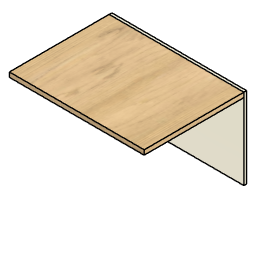
Camera mount v3 (Autodesk Fusion 360 design; units mm, degrees)
Autodesk Fusion 360 part; units mm, degrees
sketch "Sketch1" plane through (0, 0, 0) normal (0, 1, 0) x (1, 0, 0) in component "Shelf"
  line L0 (0, 0) -> (500, 0)
  line L1 (500, 0) -> (500, -17.3)
  line L2 (500, -17.3) -> (0, -17.3)
  line L3 (0, -17.3) -> (0, 0)
  line L4 (0, -17.3) -> (0, 282.7)
  line L5 (0, 282.7) -> (500, 282.7)
  line L6 (500, 282.7) -> (500, -17.3)
  dimension "d1" = 500
  dimension "d2" = 17.3
  dimension "d5" = 300
  constraint coincident L0.start L3.end
  constraint horizontal L0
  constraint perpendicular L0 L1
  constraint perpendicular L1 L2
  constraint perpendicular L0 L3
  constraint perpendicular L0 L4
  constraint perpendicular L1 L5
  constraint perpendicular L2 L6
  measures "d1" distance of L0.start L0.end
  measures "d2" distance of L0.end L1.end
  measures "d5" distance of L2.end L4.end
extrude "Extrude1" add sketch "Sketch1" against normal blind 370 contours L0 L1 L2 L3 L4 L6 makes body 1 in component "Shelf"
extrude "Extrude2" add sketch "Sketch1" along normal blind 10 separate body makes body 2 in component "Shelf"
sketch "Sketch2" plane through (0, 0, 0) normal (0, -1, 0) x (1, 0, 0) in component "Shelf"
  line L0 (0, -282.7) -> (500, -282.7)
  line L1 (500, -282.7) -> (500, 17.3)
  line L2 (500, 17.3) -> (0, 17.3)
  line L3 (0, 17.3) -> (0, -282.7)
  line L4 (0, 0) -> (500, 0)
  line L5 (500, 0) -> (0, 0)
  line L6 (236, 0) -> (236, -200)
  line L7 (236, -200) -> (264, -200)
  line L8 (264, -200) -> (264, 0)
  line L9 (250, -200) -> (250, 200) construction
  dimension "d8" = 200
  dimension "d9" = 28
  constraint coincident L5 L6.start
  constraint perpendicular L5 L6
  constraint perpendicular L6 L7
  constraint coincident L4 L8.end
  constraint perpendicular L4 L8
  constraint midpoint L7 L9.start
  constraint perpendicular L7 L9
  constraint midpoint L5 L9
  measures "d8" distance of L6.start L6.end
  measures "d9" distance of L6.end L7.end
extrude "Extrude3" add sketch "Sketch2" along normal blind 4 separate body contours L4 L5 L6 L7 L8 makes body 3 in component "Shelf"
sketch "Sketch3" plane through (0, -4, 0) normal (0, -1, 0) x (1, 0, 0) in component "Shelf"
  line L0 (264, -200) -> (264, 0)
  line L1 (264, 0) -> (236, 0)
  line L2 (236, 0) -> (236, -200)
  line L3 (236, -200) -> (264, -200)
  line L4 (236, -4) -> (264, -4)
  dimension "d12" = 4
  constraint coincident L2 L4.start
  constraint coincident L0 L4.end
  constraint perpendicular L0 L4
  measures "d12" distance of L1 L4
extrude "Extrude4" add sketch "Sketch3" along normal blind 280 contours L0 L1 L2 L4 bodies 3 in component "Shelf"
ref_plane "WorkPlane1" through (250, 0, 0) normal (1, 0, 0) x (0, 1, 0) in component "Shelf"
sketch "Sketch4" plane through (250, 0, 0) normal (1, 0, 0) x (0, 1, 0) in component "Shelf"
  line L0 (-4, -155) -> (-245.6505, -4)
  line L1 (-4, -4) -> (-284, -4)
  line L2 (-4, -4) -> (-4, -200)
  line L3 (-4, -155) -> (-186.4554, -155) construction
  line L4 (0, 0) -> (-370, 0) construction
  line L5 (-207.9089, -4) -> (-4, -131.4164)
  line L6 (-4, -131.4164) -> (-4, -155)
  line L7 (-207.9089, -4) -> (-245.6505, -4)
  dimension "d16" = 32
  dimension "d17" = 155
  dimension "d19" = 20
  constraint coincident L0.end L1
  constraint coincident L0.start L2
  constraint perpendicular L2 L3
  constraint coincident L1 L5.start
  constraint coincident L2 L5.end
  constraint parallel L0 L5
  measures "d16" angle of L0 L3
  measures "d17" distance of L0.start L4
  measures "d19" distance of L0 L5
extrude "Extrude5" add sketch "Sketch4" along normal mid plane 4.4 contours L0 L1 L2 L5 L6 L7 bodies 3 in component "Shelf"
sketch "Sketch1 (2)" plane through (247.8, 0, 0) normal (-1, 0, 0) x (0, -1, 0) in component "Mount"
  line L0 (207.9089, -4) -> (4, -131.4164)
  line L1 (4, -131.4164) -> (4, -155)
  line L2 (4, -155) -> (245.6505, -4)
  line L3 (245.6505, -4) -> (207.9089, -4)
  line L4 (0, 0) -> (0, -200)
  line L5 (0, -200) -> (4, -200)
  line L6 (4, -200) -> (4, -4)
  line L7 (4, -4) -> (284, -4)
  line L8 (284, -4) -> (284, 0)
  line L9 (284, 0) -> (0, 0)
  line L10 (4, -124.3414) -> (141.1258, -38.6557)
  line L11 (141.1258, -38.6557) -> (144.3053, -43.7439)
  dimension "d22" = 75
  dimension "d23" = 6
  constraint coincident L6 L10.start
  constraint parallel L0 L10
  constraint coincident L0 L11.end
  constraint perpendicular L0 L11
  measures "d22" distance of L0.start L11.end
  measures "d23" distance of L0 L10
sketch "Sketch5" plane through (0, -4, 0) normal (0, -1, 0) x (1, 0, 0) in component "Shelf"
  line L0 (247.8, -155) -> (247.8, -131.4164)
  line L1 (247.8, -131.4164) -> (252.2, -131.4164)
  line L2 (252.2, -131.4164) -> (252.2, -155)
  line L3 (252.2, -155) -> (247.8, -155)
  line L4 (264, -4) -> (236, -4)
  line L5 (236, -4) -> (236, -200)
  line L6 (236, -200) -> (264, -200)
  line L7 (264, -200) -> (264, -4)
  circle A0 centre (250, -188) radius 5
  line L8 (250, -155) -> (250, -197.5396) construction
  dimension "d31" = 10
  dimension "d32" = 33
  constraint midpoint L3 L8.start
  constraint perpendicular L3 L8
  constraint coincident A0.centre L8
  measures "d31" diameter of A0
  measures "d32" distance of L3 A0.centre
extrude "Extrude5'" add sketch "Sketch1 (2)" against normal blind 14.4 separate body contours L0 L6 L10 L11 makes body 4 in component "Mount"
sketch "Sketch6" plane through (262.2, 0, 0) normal (1, 0, 0) x (0, 1, 0) in component "Mount"
  line L0 (-4, -124.3414) -> (-141.1258, -38.6557)
  line L1 (-141.1258, -38.6557) -> (-144.3053, -43.7439)
  line L2 (-144.3053, -43.7439) -> (-4, -131.4164)
  line L3 (-4, -131.4164) -> (-4, -124.3414)
  line L4 (-4, -131.4164) -> (-4, -156.4164)
  line L5 (-4, -155) -> (-245.6505, -4)
  line L6 (-14, -148.7513) -> (-14, -176.9164)
  line L7 (-4, -200) -> (-4, -4)
  line L8 (-14, -176.9164) -> (-4, -176.9164)
  line L9 (-14, -148.7513) -> (-14, -125.1677)
  line L10 (-144.3053, -43.7439) -> (-155.9635, -62.401)
  line L11 (-155.9635, -62.401) -> (-14, -151.1097)
  dimension "d43" = 25
  dimension "d44" = 10
  dimension "d46" = 20.5
  dimension "d79" = 22
  constraint coincident L2.end L3.start
  constraint parallel L3 L4
  constraint coincident L5 L6.start
  constraint parallel L4 L6
  constraint coincident L7 L8.end
  constraint perpendicular L7 L8
  constraint coincident L2 L9.end
  constraint parallel L6 L9
  constraint coincident L1.end L2.start
  constraint perpendicular L5 L10
  constraint coincident L6 L11.end
  constraint perpendicular L10 L11
  measures "d43" distance of L2.end L4.end
  measures "d44" distance of L6 L7
  measures "d46" distance of L4.end L8.end
  measures "d79" distance of L1.end L10.end
extrude "Extrude6" add sketch "Sketch6" against normal blind 9.9 contours L2 L4 L5 L7 L9 | L4 L5 L6 L7 L8 bodies 4 in component "Mount"
sketch "Sketch7" plane through (0, -4, 0) normal (0, -1, 0) x (1, 0, 0) in component "Mount"
  line L0 (247.8, -155) -> (247.8, -131.4164)
  line L1 (247.8, -131.4164) -> (252.2, -131.4164)
  line L2 (252.2, -131.4164) -> (252.2, -155)
  line L3 (252.2, -155) -> (247.8, -155)
  line L4 (264, -4) -> (236, -4)
  line L5 (236, -4) -> (236, -200)
  line L6 (236, -200) -> (264, -200)
  line L7 (264, -200) -> (264, -4)
  circle A0 centre (250, -188) radius 3.5
  line L8 (250, -155) -> (250, -238.8329) construction
  line L9 (262.2, -176.9164) -> (252.3, -176.9164)
  line L10 (262.2, -176.9164) -> (262.2, -196.9164)
  line L11 (262.2, -196.9164) -> (237.8, -196.9164)
  line L12 (237.8, -196.9164) -> (237.8, -176.9164)
  line L13 (237.8, -176.9164) -> (252.3, -176.9164)
  dimension "d49" = 7
  dimension "d50" = 33
  dimension "d51" = 20
  constraint midpoint L3 L8.start
  constraint perpendicular L6 L8
  constraint coincident A0.centre L8
  constraint coincident L9.start L10.start
  constraint perpendicular L9 L10
  constraint perpendicular L10 L11
  constraint perpendicular L9 L12
  constraint coincident L9.end L13.end
  constraint perpendicular L8 L13
  constraint midpoint L8 L11
  measures "d49" diameter of A0
  measures "d50" distance of L3 A0.centre
  measures "d51" distance of L9.start L10.end
extrude "Extrude7" add sketch "Sketch7" along normal blind 6 contours L9 L10 L11 L12 L13 bodies 4 in component "Mount"
extrude "Extrude8" add 1 faces at (247.8, -50.7684, -99.8339) along direction (-1, 0, 0) blind 30 on bodies 4 bodies 4 in component "Mount"
sketch "Sketch8" plane through (217.8, 0, 0) normal (-1, 0, 0) x (0, -1, 0) in component "Mount"
  line L0 (141.1258, -38.6557) -> (4, -124.3414)
  line L1 (4, -124.3414) -> (4, -131.4164)
  line L2 (4, -131.4164) -> (144.3053, -43.7439)
  line L3 (144.3053, -43.7439) -> (141.1258, -38.6557)
  line L4 (104, -68.9295) -> (204, -68.9295) construction
  line L5 (104, -68.9295) -> (164, -68.9295)
  line L6 (164, -68.9295) -> (164, -143.9295)
  line L7 (104, -68.9295) -> (104, -143.9295)
  line L8 (104, -143.9295) -> (164, -143.9295)
  line L9 (154, -68.9295) -> (154, -165.7492) construction
  line L10 (4, -4) -> (4, -200)
  circle A0 centre (154, -133.9295) radius 3.25
  line L11 (144.3053, -43.7439) -> (164, -68.9295)
  line L12 (4, -131.4164) -> (4, -143.9295)
  line L13 (4, -143.9295) -> (104, -143.9295)
  dimension "d56" = 100
  dimension "d57" = 60
  dimension "d58" = 75
  dimension "d59" = 50
  dimension "d60" = 100
  dimension "d61" = 6.5
  dimension "d63" = 65
  constraint coincident L2 L4.start
  constraint horizontal L4
  constraint parallel L4 L5
  constraint perpendicular L4 L6
  constraint perpendicular L5 L7
  constraint perpendicular L6 L8
  constraint coincident L4 L9.start
  constraint perpendicular L8 L9
  constraint coincident L9 A0.centre
  constraint coincident L2.end L3.start
  constraint coincident L1.end L2.start
  constraint perpendicular L7 L13
  constraint perpendicular L12 L13
  measures "d56" distance of L4.start L4.end
  measures "d57" distance of L4.start L5.end
  measures "d58" distance of L5.end L6.end
  measures "d59" distance of L7 L9
  measures "d60" distance of L4.start L10
  measures "d61" diameter of A0
  measures "d63" distance of L5 A0.centre
extrude "Extrude9" add sketch "Sketch8" against normal blind 13 contours L2 L5 L11 | L2 L7 L10 L12 L13 | L5 L6 L7 L8 bodies 4 in component "Mount"
extrude "Extrude10" add 1 faces at (259.287, -10, -187.1037) along direction (0, -1, 0) blind 4 on bodies 4 bodies 4 in component "Mount"
hole "Hole1" at (250, -14, -188) direction (0, 1, 0) diameter 7 depth 10 tip angle 118 countersink diameter 10 countersink angle 80 bodies 4 in component "Mount"
fillet "Fillet1" radius 8 2 edges at (224.3, -164, -68.9295) (224.3, -164, -143.9295) on bodies 4 in component "Mount"
fillet "Fillet2" radius 3 2 edges at (240, -141.1258, -38.6557) (246.5, -144.3053, -43.7439) on bodies 4 in component "Mount"
extrude "Extrude6'" cut sketch "Sketch5" against normal blind 80 contours A0 bodies 2 3 in component "Shelf"
component "Shelf" placed x (1, 0, 0) y (0, 1, 0) z (0, 0, 1) at (0, 0, 0)
component "Mount" placed x (1, 0, 0) y (0, 1, 0) z (0, 0, 1) at (0, 0, 0)
named bodies: "Shelf", "Wall", "Bracket"
